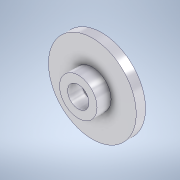
# Autodesk Inventor part: orczyk serwa okrągły 02-2
Saved by Autodesk Inventor 2021 (Build 250183000, 183)
## iProperties
Created: 2021-11-05
Part Number: orczyk serwa okrągły 02-2
Material: Generic
Document SubType Name: Modeling
Designer: Łukasz
Density: 1 g/cm^3
Appearance: Opal
Author: Łukasz
Autodesk Inventor part; units mm, degrees
ref_plane "YZ Plane" through (0, 0, 0) normal (1, 0, 0) x (0, 1, 0)
ref_plane "XZ Plane" through (0, 0, 0) normal (0, 1, 0) x (-1, 0, 0)
ref_plane "XY Plane" through (0, 0, 0) normal (0, 0, 1) x (1, 0, 0)
sketch "Sketch1" plane through (0, 0, 0) normal (0, 0, 1) x (1, 0, 0)
  circle A0 centre (0, 0) radius 10.3
  circle A1 centre (0, 0) radius 1.45
  dimension "d0" = 20.6
  dimension "d7" = 2.9
  constraints: 2 centre point, 2 coincident
  measures "d0" diameter of A0
  measures "d7" diameter of A1
extrude "Extrusion1" add sketch "Sketch1" along normal blind 2.2
sketch "Sketch2" plane through (0, 0, 2.2) normal (0, 0, 1) x (1, 0, 0)
  circle A0 centre (0, 0) radius 4.4
  circle A1 centre (0, 0) radius 2.5
  dimension "d3" = 8.8
  dimension "d4" = 5
  constraints: 2 centre point, 2 coincident
  measures "d3" diameter of A0
  measures "d4" diameter of A1
extrude "Extrusion2" add sketch "Sketch2" along normal blind 3.3
body "Solid1"
